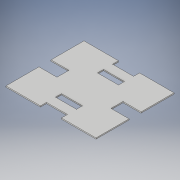
# Autodesk Inventor part: Wood Base
Saved by Autodesk Inventor 2018 (Build 220112000, 112)
## iProperties
Created: 2019-01-03
Part Number: Wood Base
Material: Generic
Document SubType Name: Modeling
Designer: Gabriel
Density: 1 g/cm^3
Appearance: Default
Author: Gabriel
Autodesk Inventor part; units mm, degrees
ref_plane "YZ Plane" through (0, 0, 0) normal (1, 0, 0) x (0, 1, 0)
ref_plane "XZ Plane" through (0, 0, 0) normal (0, 1, 0) x (-1, 0, 0)
ref_plane "XY Plane" through (0, 0, 0) normal (0, 0, 1) x (1, 0, 0)
sketch "Sketch1" plane through (0, 0, 0) normal (0, 1, 0) x (-1, 0, 0)
  line L0 (-212.3768, -1157.61) -> (-364.7768, -1157.61)
  line L1 (-364.7768, -1157.61) -> (-364.7768, -1259.21)
  line L2 (-364.7768, -1259.21) -> (-212.3768, -1259.21)
  line L3 (-974.3768, -1157.61) -> (-821.9768, -1157.61)
  line L4 (-821.9768, -1157.61) -> (-821.9768, -1259.21)
  line L5 (-821.9768, -1259.21) -> (-974.3768, -1259.21)
  line L6 (-682.2768, -929.01) -> (-504.4768, -929.01)
  line L7 (-682.2768, -1487.81) -> (-504.4768, -1487.81)
  line L8 (-504.4768, -1487.81) -> (-504.4768, -1538.61)
  line L9 (-682.2768, -1487.81) -> (-682.2768, -1538.61)
  line L10 (-504.4768, -929.01) -> (-504.4768, -878.21)
  line L11 (-682.2768, -929.01) -> (-682.2768, -878.21)
  line L12 (-504.4768, -878.21) -> (-212.3768, -878.21)
  line L13 (-212.3768, -878.21) -> (-212.3768, -1157.61)
  line L14 (-504.4768, -1538.61) -> (-212.3768, -1538.61)
  line L15 (-212.3768, -1538.61) -> (-212.3768, -1259.21)
  line L16 (-682.2768, -1538.61) -> (-974.3768, -1538.61)
  line L17 (-974.3768, -1538.61) -> (-974.3768, -1259.21)
  line L18 (-682.2768, -878.21) -> (-974.3768, -878.21)
  line L19 (-974.3768, -878.21) -> (-974.3768, -1157.61)
  line L20 (-504.4768, -1005.21) -> (-682.2768, -1005.21)
  line L21 (-682.2768, -1005.21) -> (-682.2768, -1056.01)
  line L22 (-682.2768, -1056.01) -> (-504.4768, -1056.01)
  line L23 (-504.4768, -1056.01) -> (-504.4768, -1005.21)
  line L24 (-504.4768, -1411.61) -> (-682.2768, -1411.61)
  line L25 (-682.2768, -1411.61) -> (-682.2768, -1360.81)
  line L26 (-682.2768, -1360.81) -> (-504.4768, -1360.81)
  line L27 (-504.4768, -1360.81) -> (-504.4768, -1411.61)
  dimension "d9" = 152.4
  dimension "d10" = 101.6
  dimension "d14" = 152.4
  dimension "d15" = 101.6
  dimension "d27" = 177.8
  dimension "d29" = 177.8
  dimension "d30" = 50.8
  dimension "d31" = 50.8
  dimension "d32" = 50.8
  dimension "d33" = 76.2
  dimension "d34" = 177.8
  dimension "d35" = 50.8
  dimension "d36" = 76.2
  dimension "d37" = 177.8
  dimension "d38" = 50.8
  constraints: 56 end point, 8 perpendicular, 5 horizontal, 4 parallel, 4 vertical, 1 point on line
  measures "d9" distance of L0.start L0.end
  measures "d10" distance of L0.end L1.end
  measures "d14" distance of L3.start L3.end
  measures "d15" distance of L3.end L4.end
  measures "d27" distance of L6.start L6.end
  measures "d29" distance of L7.start L7.end
  measures "d30" distance of L7.end L8.end
  measures "d31" distance of L7.start L9.end
  measures "d32" distance of L6.end L10.end
  measures "d33" distance of L6.end L20.start
  measures "d34" distance of L22.end L21.end
  measures "d35" distance of L21.end L20.end
  measures "d36" distance of L7.end L24.start
  measures "d37" distance of L25.end L26.end
  measures "d38" distance of L24.end L25.end
extrude "Extrusion3" add sketch "Sketch1" along normal blind 9.525
body "Solid3"
